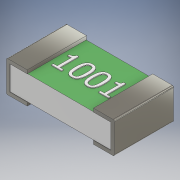
# Autodesk Inventor part: 21-1001
Saved by Autodesk Inventor 2018 (Build 220112000, 112)
## iProperties
Created: 2019-09-21
Part Number: 21-1001
Material: Copper
Document SubType Name: Modeling
Designer: Bradley
Density: 8.94 g/cm^3
Appearance: Smooth - White
Author: Bradley
Autodesk Inventor part; units mm, degrees
ref_plane "YZ Plane" through (0, 0, 0) normal (1, 0, 0) x (0, 1, 0)
ref_plane "XZ Plane" through (0, 0, 0) normal (0, 1, 0) x (-1, 0, 0)
ref_plane "XY Plane" through (0, 0, 0) normal (0, 0, 1) x (1, 0, 0)
sketch "Sketch1" plane through (0, 0, 0) normal (0, 1, 0) x (-1, 0, 0)
  line L0 (0.725, 0.175) -> (-0.725, 0.175)
  line L1 (-0.725, 0.175) -> (-0.725, -0.175)
  line L2 (-0.725, -0.175) -> (0.725, -0.175)
  line L3 (0.725, -0.175) -> (0.725, 0.175)
  line L4 (0.475, 0.175) -> (0.475, 0.225)
  line L5 (0.475, 0.225) -> (0.775, 0.225)
  line L6 (0.775, 0.225) -> (0.775, -0.225)
  line L7 (0.775, -0.225) -> (0.475, -0.225)
  line L8 (0.475, -0.225) -> (0.475, -0.175)
  line L9 (-0.475, 0.175) -> (-0.475, 0.225)
  line L10 (-0.475, 0.225) -> (-0.775, 0.225)
  line L11 (-0.775, 0.225) -> (-0.775, -0.225)
  line L12 (-0.775, -0.225) -> (-0.475, -0.225)
  line L13 (-0.475, -0.175) -> (-0.475, -0.225)
  line L14 (0.475, 0.175) -> (-0.475, 0.175)
  point P0 (0, 0)
  point P1 (0, 0.175)
  point P2 (0.725, 0)
  dimension "d0" = 1.55
  dimension "d1" = 0.05
  dimension "d2" = 0.05
  dimension "d3" = 0.45
  dimension "d4" = 0.3
  constraints: 30 end point, 12 point on line, 7 perpendicular, 3 collinear, 3 midpoint, 2 parallel, 1 horizontal, 1 horizontal alignment, 1 vertical, 1 vertical alignment
  measures "d0" distance between parallel lines of L11 L6
  measures "d1" distance of L7.end L8.end
  measures "d2" distance between parallel lines of L6 L3
  measures "d3" distance of L5.end L6.end
  measures "d4" distance of L6.end L7.end
extrude "Extrusion1" add sketch "Sketch1" along normal mid plane 0.85 contours L0 L4 L5 L6 L7 L8 L2 L3 | L0 L1 L2 L13 L12 L11 L10 L9
extrude "Extrusion2" add sketch "Sketch1" along normal mid plane 0.84 contours L3 L2 L1 L0
sketch "Sketch2" plane through (-0.475, -0.42, 0.175) normal (0, 0, 1) x (1, 0, 0)
  line L0 (0, 0) -> (0, 0.84) projected
  line L1 (0.95, 0) -> (0, 0) projected
  line L2 (0.95, 0) -> (0.95, 0.84) projected
  line L3 (0, 0.84) -> (0.95, 0.84) projected
  line L4 (0, 0.42) -> (0.95, 0.42) construction
  line L5 (0.2166, 0.27) -> (0.0702, 0.27)
  line L6 (0.0702, 0.27) -> (0.0702, 0.3006)
  line L7 (0.0702, 0.3006) -> (0.1247, 0.3006)
  line L8 (0.1247, 0.3006) -> (0.1247, 0.5017)
  line L9 (0.1247, 0.5017) -> (0.0702, 0.5017)
  line L10 (0.0702, 0.5017) -> (0.0702, 0.5292)
  spline S0 degree 2 poles (0.0702, 0.5292) (0.1011, 0.5292) (0.1303, 0.5467) (0.1322, 0.571) knots 0 0 0 1 2 2 2
  line L11 (0.1322, 0.571) -> (0.1633, 0.571)
  line L12 (0.1633, 0.571) -> (0.1633, 0.3006)
  line L13 (0.1633, 0.3006) -> (0.2166, 0.3006)
  line L14 (0.2166, 0.3006) -> (0.2166, 0.27)
  spline S1 degree 2 poles (0.4585, 0.42) (0.4585, 0.3393) (0.4115, 0.2637) (0.3627, 0.2637) knots 0 0 0 1 2 2 2
  spline S2 degree 2 poles (0.3627, 0.2637) (0.3131, 0.2637) (0.2667, 0.3407) (0.2667, 0.4198) knots 0 0 0 1 2 2 2
  spline S3 degree 2 poles (0.2667, 0.4198) (0.2667, 0.501) (0.3136, 0.5761) (0.3627, 0.5761) knots 0 0 0 1 2 2 2
  spline S4 degree 2 poles (0.3627, 0.5761) (0.412, 0.5761) (0.4585, 0.4983) (0.4585, 0.42) knots 0 0 0 1 2 2 2
  spline S5 degree 2 poles (0.4069, 0.3286) (0.4128, 0.3434) (0.4176, 0.3891) (0.4176, 0.42) knots 0 0 0 1 2 2 2
  spline S6 degree 2 poles (0.4176, 0.42) (0.4176, 0.4509) (0.4128, 0.4963) (0.4067, 0.5117) knots 0 0 0 1 2 2 2
  spline S7 degree 2 poles (0.4067, 0.5117) (0.4006, 0.527) (0.3795, 0.5428) (0.3627, 0.5428) knots 0 0 0 1 2 2 2
  spline S8 degree 2 poles (0.3627, 0.5428) (0.3459, 0.5428) (0.3243, 0.527) (0.3179, 0.5112) knots 0 0 0 1 2 2 2
  spline S9 degree 2 poles (0.3179, 0.5112) (0.3119, 0.4959) (0.3075, 0.4492) (0.3075, 0.4198) knots 0 0 0 1 2 2 2
  spline S10 degree 2 poles (0.3075, 0.4198) (0.3075, 0.3882) (0.3114, 0.3459) (0.3177, 0.3293) knots 0 0 0 1 2 2 2
  spline S11 degree 2 poles (0.3177, 0.3293) (0.3235, 0.3138) (0.3452, 0.297) (0.3627, 0.297) knots 0 0 0 1 2 2 2
  spline S12 degree 2 poles (0.3627, 0.297) (0.3792, 0.297) (0.4009, 0.3128) (0.4069, 0.3286) knots 0 0 0 1 2 2 2
  spline S13 degree 2 poles (0.6836, 0.42) (0.6836, 0.3393) (0.6367, 0.2637) (0.5878, 0.2637) knots 0 0 0 1 2 2 2
  spline S14 degree 2 poles (0.5878, 0.2637) (0.5382, 0.2637) (0.4918, 0.3407) (0.4918, 0.4198) knots 0 0 0 1 2 2 2
  spline S15 degree 2 poles (0.4918, 0.4198) (0.4918, 0.501) (0.5387, 0.5761) (0.5878, 0.5761) knots 0 0 0 1 2 2 2
  spline S16 degree 2 poles (0.5878, 0.5761) (0.6372, 0.5761) (0.6836, 0.4983) (0.6836, 0.42) knots 0 0 0 1 2 2 2
  spline S17 degree 2 poles (0.6321, 0.3286) (0.6379, 0.3434) (0.6427, 0.3891) (0.6427, 0.42) knots 0 0 0 1 2 2 2
  spline S18 degree 2 poles (0.6427, 0.42) (0.6427, 0.4509) (0.6379, 0.4963) (0.6318, 0.5117) knots 0 0 0 1 2 2 2
  spline S19 degree 2 poles (0.6318, 0.5117) (0.6257, 0.527) (0.6046, 0.5428) (0.5878, 0.5428) knots 0 0 0 1 2 2 2
  spline S20 degree 2 poles (0.5878, 0.5428) (0.571, 0.5428) (0.5494, 0.527) (0.5431, 0.5112) knots 0 0 0 1 2 2 2
  spline S21 degree 2 poles (0.5431, 0.5112) (0.537, 0.4959) (0.5326, 0.4492) (0.5326, 0.4198) knots 0 0 0 1 2 2 2
  spline S22 degree 2 poles (0.5326, 0.4198) (0.5326, 0.3882) (0.5365, 0.3459) (0.5428, 0.3293) knots 0 0 0 1 2 2 2
  spline S23 degree 2 poles (0.5428, 0.3293) (0.5487, 0.3138) (0.5703, 0.297) (0.5878, 0.297) knots 0 0 0 1 2 2 2
  spline S24 degree 2 poles (0.5878, 0.297) (0.6043, 0.297) (0.626, 0.3128) (0.6321, 0.3286) knots 0 0 0 1 2 2 2
  line L15 (0.8919, 0.27) -> (0.7456, 0.27)
  line L16 (0.7456, 0.27) -> (0.7456, 0.3006)
  line L17 (0.7456, 0.3006) -> (0.8, 0.3006)
  line L18 (0.8, 0.3006) -> (0.8, 0.5017)
  line L19 (0.8, 0.5017) -> (0.7456, 0.5017)
  line L20 (0.7456, 0.5017) -> (0.7456, 0.5292)
  spline S25 degree 2 poles (0.7456, 0.5292) (0.7765, 0.5292) (0.8056, 0.5467) (0.8076, 0.571) knots 0 0 0 1 2 2 2
  line L21 (0.8076, 0.571) -> (0.8387, 0.571)
  line L22 (0.8387, 0.571) -> (0.8387, 0.3006)
  line L23 (0.8387, 0.3006) -> (0.8919, 0.3006)
  line L24 (0.8919, 0.3006) -> (0.8919, 0.27)
  point P0 (0.475, 0.42)
  constraints: 2 end point, 2 midpoint, 1 horizontal
extrude "Extrusion3" add sketch "Sketch2" along normal blind 0.01 contours L5 L6 L7 L8 L9 L10 S0 L11 L12 L13 L14 | S1 S2 S3 S4 | S13 S14 S15 S16 | L15 L16 L17 L18 L19 L20 S25 L21 L22 L23 L24
fillet "Fillet1" radius 0.02 4 edges at (-0.775, 0, 0.225) (-0.775, 0, -0.225) (0.775, 0, 0.225) (0.775, 0, -0.225)
equation "\"d2\" = d1"
body "Solid1"
